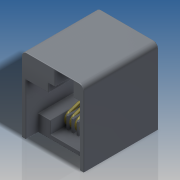
# Autodesk Inventor part: 54732b-LtBluishGray
Saved by Autodesk Inventor 2016 SP2 (Build 200236200, 236)
## iProperties
Created: 2015-08-19
Part Number: 54732b-LtBluishGray
Material: ABS Plastic
Document SubType Name: Modeling
Designer: D. Kohfeld
Density: 1.06 g/cm^3
Appearance: LtBluishGray
Mass: 1.27622 g
Surface Area: 18.8754 cm^2
Volume: 1.20398 cm^3
Author: D. Kohfeld
Autodesk Inventor part; units mm, degrees
ref_plane "XZ Plane" through (0, 0, 0) normal (0, 1, 0) x (-1, 0, 0)
ref_plane "XY Plane" through (0, 0, 0) normal (0, 0, 1) x (1, 0, 0)
sketch "Sketch2" plane through (0, 0, 0) normal (0, 0, 1) x (1, 0, 0)
  line L0 (-6, -6.8) -> (-6, 6.8)
  arc A0 (-5.04, 7.76) -> (-6, 6.8) centre (-5.04, 6.8) ccw
  line L1 (-5.04, 7.76) -> (5.04, 7.76)
  arc A1 (6, 6.8) -> (5.04, 7.76) centre (5.04, 6.8) ccw
  line L2 (6, 6.8) -> (6, -6.8)
  line L3 (6, -6.8) -> (-6, -6.8)
  line L4 (-5.2, -6.8) -> (-5.2, 3.2)
  line L5 (-5.2, 3.2) -> (-0.8, 3.2)
  line L6 (-0.8, 3.2) -> (-0.8, 4.8)
  line L7 (-0.8, 4.8) -> (0.4, 4.8)
  line L8 (0.4, 4.8) -> (0.4, 6.8)
  line L9 (0.4, 6.8) -> (4, 6.8)
  line L10 (4, 6.8) -> (4, 4.8)
  line L11 (4, 4.8) -> (5.2, 4.8)
  line L12 (5.2, 4.8) -> (5.2, -6.8)
  line L13 (-5.2, -3.6) -> (-2.8, -3.6)
  line L14 (-2.8, -3.6) -> (-2.8, -6)
  line L15 (-2.8, -6) -> (-2.2, -6)
  line L16 (-2.2, -6) -> (-1.8, -6)
  line L17 (-1.8, -6) -> (-1.2, -6)
  line L18 (-1.2, -6) -> (-0.8, -6)
  line L19 (-0.8, -6) -> (-0.2, -6)
  line L20 (-0.2, -6) -> (0.2, -6)
  line L21 (0.2, -6) -> (0.8, -6)
  line L22 (0.8, -6) -> (1.2, -6)
  line L23 (1.2, -6) -> (1.8, -6)
  line L24 (1.8, -6) -> (2.2, -6)
  line L25 (2.2, -6) -> (2.8, -6)
  line L26 (2.8, -6) -> (2.8, -3.6)
  line L27 (2.8, -3.6) -> (5.2, -3.6)
  line L28 (-2.2, -6) -> (-2.2, -3.6)
  line L29 (-1.8, -6) -> (-1.8, -3.6)
  line L30 (-1.2, -6) -> (-1.2, -3.6)
  line L31 (-0.8, -6) -> (-0.8, -3.6)
  line L32 (-0.2, -6) -> (-0.2, -3.6)
  line L33 (0.2, -6) -> (0.2, -3.6)
  line L34 (0.8, -6) -> (0.8, -3.6)
  line L35 (1.2, -6) -> (1.2, -3.6)
  line L36 (1.8, -6) -> (1.8, -3.6)
  line L37 (2.2, -6) -> (2.2, -3.6)
  line L38 (-2.8, -3.6) -> (-2.2, -3.6)
  line L39 (-2.2, -3.6) -> (-1.8, -3.6)
  line L40 (-1.8, -3.6) -> (-1.2, -3.6)
  line L41 (-1.2, -3.6) -> (-0.8, -3.6)
  line L42 (-0.8, -3.6) -> (-0.2, -3.6)
  line L43 (-0.2, -3.6) -> (0.2, -3.6)
  line L44 (0.2, -3.6) -> (0.8, -3.6)
  line L45 (0.8, -3.6) -> (1.2, -3.6)
  line L46 (1.2, -3.6) -> (1.8, -3.6)
  line L47 (1.8, -3.6) -> (2.2, -3.6)
  line L48 (2.2, -3.6) -> (2.8, -3.6)
  line L49 (-0.8, 4.8) -> (-0.8, 6.8)
  line L50 (-0.8, 6.8) -> (0.4, 6.8)
  line L51 (4, 6.8) -> (5.2, 6.8)
  line L52 (5.2, 6.8) -> (5.2, 4.8)
  point P0 (0, 0)
  point P1 (0, 7.76)
  point P2 (-6, 0)
  dimension "d0" = 12
  dimension "d1" = 14.56
  dimension "d2" = 0.96
  dimension "d3" = 10.4
  dimension "d4" = 0.96
  dimension "d5" = 3.6
  dimension "d6" = 6
  dimension "d8" = 2
  dimension "d9" = 1.6
  dimension "d10" = 0.8
  dimension "d11" = 3.2
  dimension "d12" = 2.4
  dimension "d13" = 0.4
  dimension "d14" = 5.6
  constraints: 106 end point, 32 horizontal, 21 vertical, 11 collinear, 4 point on circle, 4 point on line, 4 tangent, 2 centre point, 2 horizontal alignment, 2 midpoint, 1 equal radius, 1 vertical alignment
  measures "d0" distance between parallel lines of L0 L2
  measures "d1" distance between parallel lines of L3 L1
  measures "d2" radius of A0
  measures "d3" distance between parallel lines of L12 L4
  measures "d4" distance between parallel lines of L1 L9
  measures "d5" distance of L8.end L9.end
  measures "d6" distance between parallel lines of L12 L6
  measures "d8" distance of L7.end L8.end
  measures "d9" distance of L5.end L6.end
  measures "d10" distance between parallel lines of L0 L4
  measures "d11" distance between parallel lines of L3 L13
  measures "d12" distance of L13.end L14.end
  measures "d13" distance between parallel lines of L29 L28
  measures "d14" distance between parallel lines of L26 L14
extrude "Extrusion1" add sketch "Sketch2" against normal blind 14.4
extrude "Extrusion2" cut sketch "Sketch2" against normal blind 12.8 contours L4 L5 L6 L7 L8 L9 L10 L11 L12 L27 L48 L47 L46 L45 L44 L43 L42 L41 L40 L39 L38 L13 | L11 L10 L51 L52 | L49 L50 L8 L7
extrude "Extrusion3" add sketch "Sketch2" against normal blind 2.8 contours L11 L10 L51 L52 | L49 L50 L8 L7
extrude "Extrusion4" cut sketch "Sketch2" against normal blind 9.6 contours L38 L28 L15 L14 | L26 L25 L37 L48 | L40 L30 L17 L29 | L36 L23 L35 L46 | L42 L32 L19 L31 | L34 L21 L33 L44
extrude "Extrusion5" cut sketch "Sketch2" against normal blind 2.4 contours L4 L13 L14 L15 L16 L17 L18 L19 L20 L21 L22 L23 L24 L25 L26 L27 L12 L3 | L39 L29 L16 L28 | L37 L24 L36 L47 | L41 L31 L18 L30 | L35 L22 L34 L45 | L43 L33 L20 L32
extrude "Extrusion6" cut sketch "Sketch2" against normal blind 4.8 contours L39 L29 L16 L28 | L37 L24 L36 L47 | L41 L31 L18 L30 | L35 L22 L34 L45 | L43 L33 L20 L32
sketch "Sketch3" plane through (0, 0, -9.6) normal (0, 0, 1) x (1, 0, 0)
  line L0 (-2.2, -6) -> (-2.8, -6) projected
  circle A0 centre (-2.5, -5.71) radius 0.29
  line L1 (-2.8, -6) -> (2.8, -6) projected
  point P0 (0, 0)
  point P1 (-2.5, -6)
  dimension "d27" = 0.58
  constraints: 1 centre point, 1 midpoint, 1 tangent, 1 vertical alignment
  measures "d27" diameter of A0
ref_plane "Work Plane1" through (-2.5, -5.71, -9.6) normal (1, 0, 0) x (0, 1, 0)
sketch "Sketch4" plane through (-2.5, -5.71, -9.6) normal (1, 0, 0) x (0, 1, 0)
  line L0 (-0.29, 4.8) -> (2.11, 4.8) projected
  line L1 (2.11, 0) -> (2.11, 4.8) projected
  line L2 (0, 0) -> (0, 3.51)
  arc A0 (1.9509, 3.8195) -> (0, 3.51) centre (1, 3.51) ccw
  line L3 (1.9509, 3.8195) -> (3.91, -2.2)
  line L4 (-0.29, 0) -> (2.11, 0) projected
  point P0 (5.71, 9.6)
  dimension "d28" = 0.29
  dimension "d29" = 1
  dimension "d31" = 1.8
  dimension "d32" = 2.2
  constraints: 4 end point, 2 point on circle, 2 tangent, 1 centre point, 1 vertical
  measures "d28" distance edge to line of A0 L0
  measures "d29" radius of A0
  measures "d31" distance from line of L3.end L1
  measures "d32" distance from line of L3.end L4
sweep "Sweep1" add profiles "Sketch3" path "Sketch4" path curves L2 A0 L3
pattern_linear "Rectangular Pattern1" count 6 spacing 1 along (1, 0, 0) of "Sweep1"
sketch "Sketch5" plane through (0.4, 4.8, 0) normal (1, 0, 0) x (0, 0, -1)
  line L0 (0, 2) -> (2.8, 2) projected
  line L1 (0, 2) -> (0, 2.8)
  line L2 (0, 2.8) -> (2.8, 2)
  point P0 (0, -4.8)
  dimension "d37" = 0.8
  constraints: 4 end point, 1 vertical
  measures "d37" distance of L0.start L1.end
extrude "Extrusion7" cut sketch "Sketch5" along normal blind 3.6
fillet "Fillet1" radius 0.1 25 edges at (-4, -3.6, -2.4) (-2.8, -3.6, -6) (-2.8, -4.8, -2.4) (0, -6, -2.4) (-2, -3.6, -4.8) (-1, -3.6, -4.8) (0, -3.6, -4.8) (1, -3.6, -4.8) (2, -3.6, -4.8) (4, -3.6, -2.4) (2.8, -3.6, -6) (2.8, -4.8, -2.4) (5.2, -1, 0) (4.6, 4.8, 0) (4, 4.8, -1.4) (4, 6.2, 0) (2.2, 7.6, 0) (0.4, 6.2, 0) (-0.2, 4.8, 0) (0.4, 4.8, -1.4) (-0.8, 4, 0) (-0.8, 3.2, -6.4) (-3, 3.2, 0) (-5.2, -1.8, 0) (2.2, 6.8, -2.8)
fillet "Fillet2" radius 0.1 20 edges at (-5.7188, 7.4788, 0) (-6, 0, 0) (5.7188, 7.4788, 0) (6, 0, 0) (0, 7.76, 0) (-5.2, -6.8, -1.25) (-5.65, -6.8, 0) (-5.2293, -6.8, -0.0293) (5.2293, -6.8, -0.0293) (5.2, -6.8, -1.25) (5.65, -6.8, 0) (6, -6.8, -7.2) (5.7188, 7.4788, -14.4) (0, 7.76, -14.4) (-5.7188, 7.4788, -14.4) (-6, 0, -14.4) (6, 0, -14.4) (0, -6.8, -14.4) (0, -6.8, -2.4) (-6, -6.8, -7.2)
equation "\"d21\" = lh"
equation "\"d28\" = 0.5 * d27"
equation "\"lh\" = 9.6"
body "Solid1"
